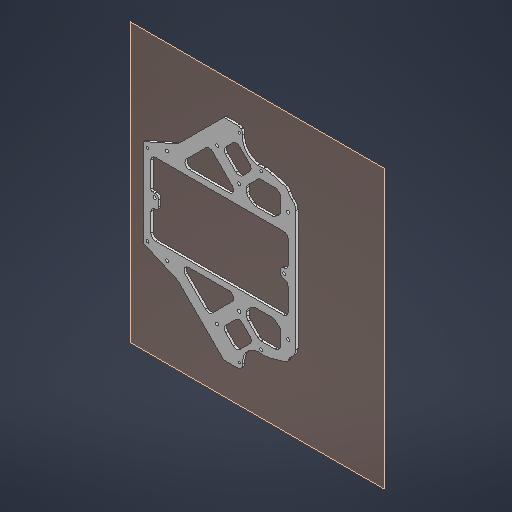
# Autodesk Inventor part: NewBody
Saved by Autodesk Inventor 2026.1 (Build 301233020, 233B)
## iProperties
Created: 2026-01-11
Part Number: NewBody
Material: 一般
Document SubType Name: Modeling
Designer: kamada
Density: 1 g/cm^3
Appearance: 既定
Author: kamada
Autodesk Inventor part; units mm, degrees
(part 1 of 2)
ref_plane "YZ Plane" through (0, 0, 0) normal (1, 0, 0) x (0, 1, 0)
ref_plane "XZ Plane" through (0, 0, 0) normal (0, 1, 0) x (-1, 0, 0)
ref_plane "XY Plane" through (0, 0, 0) normal (0, 0, 1) x (1, 0, 0)
ref_plane "作業平面1" through (0, 0, 0) normal (0, 0, 1) x (1, 0, 0)
sketch "スケッチ1" plane through (0, 0, 0) normal (0, 0, 1) x (1, 0, 0)
  line L0 (95, 63.3506) -> (95, -15.777) projected
  ellipse E0 centre (89, -15.777) end of major axis (89, -21.777) minor radius 6 (93.618, -19.6078) -> (95, -15.777) ccw projected
  ellipse E1 centre (89, -15.777) end of major axis (83, -15.777) minor radius 6 (92.5, -20.6504) -> (93.618, -19.6078) ccw projected
  ellipse E2 centre (96, -25.5238) end of major axis (90, -25.5238) minor radius 6 (92.5, -20.6504) -> (90, -25.5238) ccw projected
  line L1 (90, -40.6801) -> (90, -25.5238) projected
  line L2 (71.7064, -58.9737) -> (90, -40.6801) projected
  line L3 (61.6653, -58.9737) -> (71.7064, -58.9737) projected
  line L4 (7.6928, -5.0012) -> (61.6653, -58.9737) projected
  circle A0 centre (43.3868, -26.8548) radius 1.05 projected
  circle A1 centre (57.8825, -12.3591) radius 1.05 projected
  circle A2 centre (72.5196, -26.9962) radius 1.05 projected
  circle A3 centre (57.8825, 59.9352) radius 1.05 projected
  circle A4 centre (43.3868, 74.4309) radius 1.05 projected
  circle A5 centre (72.5196, 74.5724) radius 1.05 projected
  ellipse E3 centre (89, 63.3506) end of major axis (89, 69.3506) minor radius 6 (95, 63.3506) -> (92.5, 68.224) ccw projected
  ellipse E4 centre (96, 73.0974) end of major axis (96, 79.0974) minor radius 6 (90, 73.0974) -> (92.5, 68.224) ccw projected
  line L5 (90, 88.2549) -> (90, 73.0974) projected
  line L6 (71.7064, 106.5485) -> (90, 88.2549) projected
  line L7 (61.6653, 106.5485) -> (71.7064, 106.5485) projected
  line L8 (7.6928, 52.576) -> (61.6653, 106.5485) projected
  line L9 (90, 52.5748) -> (-5, 52.5748) projected
  line L10 (-5, 36.1871) -> (-5, 52.5748) projected
  line L11 (-5, 32.971) -> (-5, 36.1873) projected
  line L12 (-5, 30.2874) -> (-5, 32.971) projected
  line L13 (-5, 17.2874) -> (-5, 30.2874) projected
  line L14 (-5, 14.6035) -> (-5, 17.2874) projected
  line L15 (-5, 11.3873) -> (-5, 14.6035) projected
  line L16 (-5, 11.3871) -> (-5, -5.0012) projected
  line L17 (0, -5) -> (90, -5) projected
  line L18 (7.6928, -5.0012) -> (-5, -5.0012) projected
  line L19 (53.5082, 23.0012) -> (5, 23.0012) projected
  line L20 (53.5082, 24.5012) -> (53.5082, 23.0012) projected
  ellipse E5 centre (57.0082, 24.5012) end of major axis (53.5082, 24.5012) minor radius 3.5 (60.5082, 24.5012) -> (53.5082, 24.5012) ccw projected
  line L21 (60.5082, 18.2012) -> (60.5082, 24.5012) projected
  line L22 (0, 18.2012) -> (60.5082, 18.2012) projected
  line L23 (0, 18.2012) -> (0, 0) projected
  line L24 (90, 0) -> (0, 0) projected
  line L25 (90, 0) -> (90, 47.576) projected
  line L26 (0, 47.576) -> (90, 47.576) projected
  line L27 (0, 47.576) -> (0, 28.0012) projected
  arc A6 (0, 28.0012) -> (1, 27.0012) centre (1, 28.0012) ccw projected
  line L28 (1, 27.0012) -> (2.5, 27.0012) projected
  ellipse E6 centre (2.5, 24.5012) end of major axis (5, 24.5012) minor radius 2.5 (5, 24.5012) -> (2.5, 27.0012) ccw projected
  line L29 (5, 24.5012) -> (5, 23.0012) projected
  line L30 (87, 20.7876) -> (87, 22.9055) projected
  circle A7 centre (87.471, 23.7874) radius 1 projected
  ellipse E7 centre (87.471, 23.7874) end of major axis (84.4343, 23.7874) minor radius 3.0367 (85, 22.0222) -> (87, 20.7874) ccw projected
  arc A8 (90, 17.7874) -> (87, 20.7874) centre (87, 17.7874) ccw projected
  line L31 (90, 26.7874) -> (90, 17.7874) projected
  line L32 (90, 26.7874) -> (87, 26.7874) projected
  ellipse E8 centre (87.471, 23.7874) end of major axis (84.4343, 23.7874) minor radius 3.0367 (87, 26.7874) -> (85, 25.5526) ccw projected
  line L33 (85, 22.0222) -> (85, 25.5526) projected
  ellipse E9 centre (87, 29.7874) end of major axis (87, 32.7874) minor radius 3 (87, 26.7874) -> (90, 29.7874) ccw projected
  line L34 (90, 47.5748) -> (90, 52.5748) projected
  line L35 (90, -20.2311) -> (90, 0) projected
  circle A9 centre (72.5196, 74.5724) radius 1.05 projected
  circle A10 centre (43.3868, 74.4309) radius 1.05 projected
  circle A11 centre (57.8825, 59.9352) radius 1.05 projected
  line L36 (74.0275, 76.9631) -> (69.9975, 76.6465) projected
  line L37 (69.9975, 76.6465) -> (64.2656, 70.9146) projected
  line L38 (64.2656, 70.9146) -> (47.9538, 82.5385) projected
  line L39 (47.9538, 82.5385) -> (37.0141, 71.5988) projected
  line L40 (37.0141, 71.5988) -> (55.3316, 53.2813) projected
  line L41 (55.3316, 53.2813) -> (78.0106, 76.3832) projected
  line L42 (78.0106, 76.3832) -> (74.0275, 76.9631) projected
  circle A12 centre (72.5196, -26.9962) radius 1.05 projected
  circle A13 centre (43.3868, -26.8548) radius 1.05 projected
  circle A14 centre (57.8825, -12.3591) radius 1.05 projected
  line L43 (64.2656, -23.3385) -> (47.9538, -34.9624) projected
  line L44 (70.0856, -29.1585) -> (64.2656, -23.3385) projected
  ellipse E10 centre (71.1407, -40.1131) end of major axis (82.146, -40.1131) minor radius 11.0053 (73.7648, -29.4252) -> (70.0856, -29.1585) ccw projected
  line L45 (78.0106, -28.8071) -> (73.7648, -29.4252) projected
  line L46 (55.3316, 53.2813) -> (85.5, 84.0122) projected
  line L47 (85.5, 84.0122) -> (85.5, 88.2549) projected
  line L48 (85.5, 88.2549) -> (71.7064, 102.0485) projected
  line L49 (71.7064, 102.0485) -> (67.4638, 102.0485) projected
  line L50 (67.4638, 102.0485) -> (37.0141, 71.5988) projected
  arc A15 (90, -13.4106) -> (90, -11.3106) centre (89.9988, -12.3606) ccw projected
  line L51 (90, -19.6078) -> (90, -13.4106) projected
  line L52 (93.618, -19.6078) -> (90, -19.6078) projected
  ellipse E11 centre (89, -15.777) end of major axis (89, -21.777) minor radius 6 (93.618, -19.6078) -> (95, -15.777) ccw projected
  line L53 (95, 63.3506) -> (95, -15.777) projected
  ellipse E12 centre (89, 63.3506) end of major axis (89, 69.3506) minor radius 6 (95, 63.3506) -> (92.5, 68.224) ccw projected
  ellipse E13 centre (96, 73.0974) end of major axis (96, 79.0974) minor radius 6 (90, 73.0974) -> (92.5, 68.224) ccw projected
  line L54 (90, 88.2549) -> (90, 73.0974) projected
  line L55 (71.7064, 106.5485) -> (90, 88.2549) projected
  line L56 (61.6653, 106.5485) -> (71.7064, 106.5485) projected
  line L57 (7.6928, 52.576) -> (61.6653, 106.5485) projected
  line L58 (7.6928, 52.576) -> (0, 52.576) projected
  line L59 (0, 52.576) -> (0, 52.5748) projected
  line L60 (90, 52.5748) -> (0, 52.5748) projected
  line L61 (90, 47.5748) -> (90, 52.5748) projected
  line L62 (90, 29.7874) -> (90, 47.5748) projected
  ellipse E14 centre (87, 29.7874) end of major axis (87, 32.7874) minor radius 3 (87, 26.7874) -> (90, 29.7874) ccw projected
  line L63 (90, 26.7874) -> (87, 26.7874) projected
  line L64 (90, 0) -> (90, 26.7874) projected
  line L65 (0, 0) -> (90, 0) projected
  line L66 (0, 0) -> (0, -5) projected
  line L67 (0, -5) -> (90, -5) projected
  line L68 (90, -11.3106) -> (90, -5) projected
  circle A16 centre (89.9993, 59.9351) radius 1.05 projected
  line L69 (67.4638, 102.0485) -> (37.0141, 71.5988) projected
  line L70 (71.7064, 102.0485) -> (67.4638, 102.0485) projected
  line L71 (85.5, 88.2549) -> (71.7064, 102.0485) projected
  line L72 (85.5, 84.0122) -> (85.5, 88.2549) projected
  line L73 (55.3316, 53.2813) -> (85.5, 84.0122) projected
  line L74 (37.0141, 71.5988) -> (55.3316, 53.2813) projected
  line L75 (85.5, -36.4374) -> (85.5, -40.6801) projected
  line L76 (71.7064, -54.4737) -> (67.4638, -54.4737) projected
  arc A17 (90, -11.3106) -> (90, -13.4106) centre (89.9988, -12.3606) ccw projected
  line L77 (90, -11.3106) -> (90, -5) projected
  line L78 (90, -5) -> (0, -5) projected
  line L79 (0, 0) -> (0, -5) projected
  line L80 (0, 11.3871) -> (0, 0) projected
  line L81 (0, 11.3871) -> (-5, 11.3871) projected
  line L82 (-5, 11.3871) -> (-5, -5.0012) projected
  line L83 (7.6928, -5.0012) -> (-5, -5.0012) projected
  line L84 (7.6928, -5.0012) -> (61.6653, -58.9737) projected
  line L85 (61.6653, -58.9737) -> (71.7064, -58.9737) projected
  line L86 (71.7064, -58.9737) -> (90, -40.6801) projected
  line L87 (90, -40.6801) -> (90, -25.5238) projected
  ellipse E15 centre (96, -25.5238) end of major axis (90, -25.5238) minor radius 6 (92.5, -20.6504) -> (90, -25.5238) ccw projected
  ellipse E16 centre (89, -15.777) end of major axis (83, -15.777) minor radius 6 (92.5, -20.6504) -> (93.618, -19.6078) ccw projected
  line L88 (90, -19.6078) -> (93.618, -19.6078) projected
  line L89 (90, -19.6078) -> (90, -13.4106) projected
  line L90 (-5, 36.1871) -> (0, 36.1871) projected
  line L91 (0, 36.1871) -> (0, 47.5748) projected
  line L92 (0, 47.5748) -> (90, 47.5748) projected
  line L93 (90, 47.5748) -> (90, 52.5748) projected
  line L94 (90, 52.5748) -> (-5, 52.5748) projected
  line L95 (-5, 36.1871) -> (-5, 52.5748) projected
  line L96 (53.5082, 23.0012) -> (5, 23.0012) projected
  line L97 (53.5082, 24.5012) -> (53.5082, 23.0012) projected
  ellipse E17 centre (57.0082, 24.5012) end of major axis (53.5082, 24.5012) minor radius 3.5 (60.5082, 24.5012) -> (53.5082, 24.5012) ccw projected
  line L98 (60.5082, 18.2012) -> (60.5082, 24.5012) projected
  line L99 (0, 18.2012) -> (60.5082, 18.2012) projected
  line L100 (0, 18.2012) -> (0, 0) projected
  line L101 (90, 0) -> (0, 0) projected
  line L102 (90, 0) -> (90, 47.576) projected
  line L103 (0, 47.576) -> (90, 47.576) projected
  line L104 (0, 47.576) -> (0, 28.0012) projected
  arc A18 (0, 28.0012) -> (1, 27.0012) centre (1, 28.0012) ccw projected
  line L105 (1, 27.0012) -> (2.5, 27.0012) projected
  ellipse E18 centre (2.5, 24.5012) end of major axis (5, 24.5012) minor radius 2.5 (5, 24.5012) -> (2.5, 27.0012) ccw projected
  line L106 (5, 24.5012) -> (5, 23.0012) projected
  line L107 (-5, 36.1871) -> (0, 36.1871) projected
  line L108 (0, 36.1871) -> (0, 47.5748) projected
  line L109 (0, 47.5748) -> (90, 47.5748) projected
  line L110 (90, 47.5748) -> (90, 52.5748) projected
  line L111 (90, 52.5748) -> (-5, 52.5748) projected
  line L112 (-5, 36.1871) -> (-5, 52.5748) projected
  line L113 (7.6935, 52.5766) -> (7.6916, 52.5748)
  line L114 (-5, 11.3873) -> (-5, 11.3871)
  line L115 (7.6931, -5.0015) -> (7.6916, -5)
  line L116 (67.4638, -54.4724) -> (47.9538, -34.9624) projected
  line L117 (47.9538, -34.9624) -> (37.0141, -24.0227) projected
  line L118 (37.0141, -24.024) -> (55.3316, -5.7065) projected
  line L119 (55.3316, -5.7065) -> (85.5, -36.4374) projected
  line L120 (85.5, -40.6788) -> (71.7064, -54.4724) projected
  line L121 (71.7064, -54.4724) -> (67.4638, -54.4724) projected
  point P0 (93.618, -19.6078)
  point P1 (78.0095, -28.8072)
  constraints: 6 end point, 6 point on line, 1 vertical, 20 other
extrude "押し出し1" add sketch "スケッチ1" along normal blind 1.5 contours L0 E0 L52 L35 A15 L25 L34 L9 L8 L7 L6 L5 E4 E3 | E1 E2 L1 L2 L3 L4 L17 L35 A17 L52 | L17 L66 L24 L35 | L9 L34 L26 L27 L90 L10 | L18 L16 L81 L23 L66 | A8 E7 L33 E8 L32 L25 | L81 L15 L14 L13 L12 L11 L90 L27 A6 L28 E6 L29 L19 L20 E5 L21 L22 L23 | L32 E9 L25 | L42 L41 L40 L39 L38 L37 L36 | L43 L117 L118 L119 L45 E10 L44
sketch "スケッチ2" plane through (0, 0, 1.5) normal (0, 0, 1) x (1, 0, 0)
  circle A0 centre (57.0082, 24.5003) radius 1 projected
  circle A1 centre (2.5, 24.5003) radius 1 projected
  point P0 (0, 0)
extrude "押し出し2" cut sketch "スケッチ2" against normal blind 1.5
sketch "スケッチ3" plane through (0, 0, 0) normal (0, 0, -1) x (-1, 0, 0)
  arc A0 (-57.6107, -43.5509) -> (-55.9649, -41.9051) centre (-58.0239, -41.4919) ccw projected
  line L0 (-42.9736, -28.9138) -> (-55.9649, -41.9051) projected
  arc A1 (-42.9736, -28.9138) -> (-41.3278, -27.268) centre (-43.3868, -26.8548) ccw projected
  line L1 (-40.5951, -26.5353) -> (-41.3278, -27.268) projected
  line L2 (-41.7251, -25.4053) -> (-40.5951, -26.5353) projected
  arc A2 (-41.7251, -22.5768) -> (-41.7251, -25.4053) centre (-40.3109, -23.991) ccw projected
  line L3 (-40.5951, -21.4468) -> (-41.7251, -22.5768) projected
  line L4 (-41.585, -20.4569) -> (-40.5951, -21.4468) projected
  line L5 (-60.1861, -39.058) -> (-41.585, -20.4569) projected
  arc A3 (-60.4529, -42.7372) -> (-60.1861, -39.058) centre (-71.1407, -40.1131) ccw projected
  line L6 (-58.6249, -44.5651) -> (-60.4529, -42.7372) projected
  line L7 (-57.6107, -43.5509) -> (-58.6249, -44.5651) projected
  circle A4 centre (-43.3868, -26.8548) radius 0.75 projected
  circle A5 centre (-58.0239, -41.4919) radius 0.75 projected
  line L8 (-41.585, 68.033) -> (-60.1861, 86.6341) projected
  line L9 (-40.5951, 69.0229) -> (-41.585, 68.033) projected
  line L10 (-41.7251, 70.1529) -> (-40.5951, 69.0229) projected
  arc A6 (-41.7251, 72.9814) -> (-41.7251, 70.1529) centre (-40.3109, 71.5672) ccw projected
  line L11 (-40.5951, 74.1114) -> (-41.7251, 72.9814) projected
  line L12 (-41.3278, 74.8441) -> (-40.5951, 74.1114) projected
  arc A7 (-41.3278, 74.8441) -> (-42.9736, 76.4899) centre (-43.3868, 74.4309) ccw projected
  line L13 (-55.9649, 89.4813) -> (-42.9736, 76.4899) projected
  arc A8 (-55.9649, 89.4813) -> (-57.6107, 91.127) centre (-58.0239, 89.068) ccw projected
  line L14 (-58.6249, 92.1412) -> (-57.6107, 91.127) projected
  line L15 (-60.4529, 90.3133) -> (-58.6249, 92.1412) projected
  arc A9 (-60.1861, 86.6341) -> (-60.4529, 90.3133) centre (-71.1407, 87.6892) ccw projected
  circle A10 centre (-58.0239, 89.068) radius 0.75 projected
  circle A11 centre (-43.3868, 74.4309) radius 0.75 projected
  line L16 (-86.7048, 88.7216) -> (-68.878, 106.5485) projected
  line L17 (-86.7048, 77.1384) -> (-86.7048, 88.7216) projected
  line L18 (-79.7466, 78.1515) -> (-86.7048, 77.1384) projected
  line L19 (-79.7466, 78.1515) -> (-85.5, 84.0122) projected
  line L20 (-85.5, 84.0122) -> (-85.5, 88.2549) projected
  line L21 (-85.5, 88.2549) -> (-71.7064, 102.0485) projected
  line L22 (-71.7064, 102.0485) -> (-67.4638, 102.0485) projected
  line L23 (-67.4638, 102.0485) -> (-47.9538, 82.5385) projected
  line L24 (-47.9538, 82.5385) -> (-41.9405, 86.8236) projected
  line L25 (-41.9405, 86.8236) -> (-61.6653, 106.5485) projected
  line L26 (-61.6653, 106.5485) -> (-68.878, 106.5485) projected
  line L27 (-64.2656, 70.9146) -> (-41.9405, 86.8236) projected
  line L28 (-69.9975, 76.6465) -> (-64.636, 71.2849) projected
  line L29 (-64.2656, -23.3378) -> (-41.9405, -39.2473) projected
  line L30 (-68.878, -58.9724) -> (-86.7056, -41.1448) projected
  line L31 (-61.6653, -58.9724) -> (-68.878, -58.9724) projected
  line L32 (-41.9405, -39.2475) -> (-61.6653, -58.9724) projected
  line L33 (-41.9405, -39.2475) -> (-47.9538, -34.9624) projected
  line L34 (-67.4638, -54.4724) -> (-47.9538, -34.9624) projected
  line L35 (-71.7064, -54.4724) -> (-67.4638, -54.4724) projected
  line L36 (-85.5, -40.6788) -> (-71.7064, -54.4724) projected
  line L37 (-85.5, -36.4361) -> (-85.5, -40.6788) projected
  line L38 (-79.7466, -30.5754) -> (-85.5, -36.4361) projected
  line L39 (-86.7056, -29.5622) -> (-79.7466, -30.5754) projected
  line L40 (-86.7056, -41.1448) -> (-86.7056, -29.5622) projected
  line L41 (-60.4529, -42.7372) -> (-58.0907, -45.0993)
  line L42 (-64.636, -23.7082) -> (-64.2656, -23.3378)
  line L43 (-60.4529, 90.3133) -> (-58.0907, 92.6754)
  line L44 (-64.636, 71.2849) -> (-64.2656, 70.9146)
  line L45 (-64.636, 71.2849) -> (-54.3661, 80.8141)
  line L46 (-64.636, -23.7082) -> (-54.7361, -33.608)
  line L47 (-60.3757, -39.2475) -> (-54.7361, -33.608)
  line L48 (-54.7361, -33.608) -> (-64.636, -23.7082)
  line L49 (-70.2755, -29.3477) -> (-60.3757, -39.2475)
  line L50 (-67.4638, -54.4724) -> (-47.9538, -34.9624) projected
  line L51 (-47.9538, -34.9624) -> (-64.2656, -23.3385) projected
  line L52 (-60.1861, -39.058) -> (-52.7049, -31.5767)
  line L53 (-52.7049, -31.5767) -> (-62.6047, -21.6769)
  line L54 (-70.086, -29.1582) -> (-60.1861, -39.058)
  line L55 (-70.0856, -29.1585) -> (-64.2656, -23.3385) projected
  line L56 (-69.9975, 76.6465) -> (-60.1861, 86.6341)
  point P0 (0, 0)
  constraints: 26 end point, 9 point on line, 4 perpendicular, 3 parallel, 1 collinear, 1 point on circle
extrude "押し出し3" add sketch "スケッチ3" against normal up to surface (1.5 mm away) contours L7 L6 A3 L5 L29 L0 A0 | A0 L0 L29 L34 L41 L7 | L5 L46 L42 L29 | L54 L55 L46 L5 | L45 L28 L56 L8 | L8 A9 L15 L14 A8 L13 L27 | L8 L27 L44 L45 | L13 A8 L14 L43 L23 L27
sketch "スケッチ4" plane through (0, 0, 0) normal (0, 0, -1) x (-1, 0, 0)
  circle A0 centre (-71.1407, -40.1131) radius 10 projected
  circle A1 centre (-71.1407, 87.6892) radius 10 projected
  ellipse E0 centre (-71.1407, -40.1131) end of major axis (-60.1355, -40.1131) minor radius 11.0053 (-70.0856, -29.1585) -> (-73.7648, -29.4252) ccw projected
  circle A2 centre (-71.1407, -40.1131) radius 11.0053
  line L0 (-70.0856, -29.1585) -> (-60.1861, -39.058) projected
  line L1 (-60.1861, 86.6341) -> (-69.9975, 76.6465) projected
  circle A3 centre (-71.1407, -40.1131) radius 11.0053
  circle A4 centre (-71.1407, 87.6892) radius 11.1017
  line L2 (-60.1861, 86.6341) -> (-60.0794, 86.7428)
  arc A5 (-60.1861, 86.6341) -> (-60.4529, 90.3133) centre (-71.1407, 87.6892) ccw projected
  line L3 (-58.0907, 92.6754) -> (-60.4529, 90.3133) projected
  point P0 (0, 0)
  point P1 (-68.6682, 77.9997)
  point P2 (-61.4087, 85.3896)
  point P3 (-60.3732, 90.3929)
  constraints: 3 coincident, 3 point on circle, 2 centre point, 2 end point, 4 other
extrude "押し出し4" cut sketch "スケッチ4" against normal up to surface (1.5 mm away) contours L0 A0 | A0 L0 A2 | L1 A1 | A1 L1 L2 A4 | A5 L3 A4 L2 picked at (-64.1383, -34.6551) picked at (-65.57, 80.7173)
fillet "フィレット1" radius 3 4 edges at (0, 47.576, 0.75) (0, 0, 0.75) (90, 47.576, 0.75) (90, 0, 0.75)
sketch "スケッチ5" plane through (0, 0, 0) normal (0, 0, -1) x (-1, 0, 0)
  circle A0 centre (-72.5196, -26.9962) radius 1.05 projected
  circle A1 centre (-58.0239, -41.4919) radius 0.75 projected
  circle A2 centre (-43.3868, -26.8548) radius 1.05 projected
  circle A3 centre (-57.8825, -12.3591) radius 1.05 projected
  circle A4 centre (-72.5196, 74.5724) radius 1.05 projected
  circle A5 centre (-57.8825, 59.9352) radius 1.05 projected
  circle A6 centre (-43.3868, 74.4309) radius 1.05 projected
  circle A7 centre (-58.0239, 89.068) radius 0.75 projected
  line L0 (-72.5196, -26.9962) -> (-58.0239, -41.4919)
  line L1 (-58.0239, -41.4919) -> (-43.3868, -26.8548)
  line L2 (-43.3868, -26.8548) -> (-57.8825, -12.3591)
  line L3 (-57.8825, -12.3591) -> (-72.5196, -26.9962)
  line L4 (-72.5196, 74.5724) -> (-58.0239, 89.068)
  line L5 (-58.0239, 89.068) -> (-43.3868, 74.4309)
  line L6 (-43.3868, 74.4309) -> (-57.8825, 59.9352)
  line L7 (-57.8825, 59.9352) -> (-72.5196, 74.5724)
  line L8 (-67.0029, 72.5912) -> (-57.8825, 63.4708)
  line L9 (-57.8825, 63.4708) -> (-46.9223, 74.4309)
  line L10 (-46.9223, 74.4309) -> (-56.0428, 83.5514)
  line L11 (-56.0428, 83.5514) -> (-67.0029, 72.5912)
  arc A8 (-69.9975, 76.6465) -> (-60.3732, 90.3929) centre (-71.1407, 87.6892) ccw projected
  line L12 (-65.2717, -34.2441) -> (-50.6346, -19.607)
  line L13 (-56.111, -36.0435) -> (-67.0711, -25.0833)
  line L14 (-67.0711, -25.0833) -> (-57.8825, -15.8947)
  line L15 (-57.8825, -15.8947) -> (-46.9223, -26.8548)
  line L16 (-46.9223, -26.8548) -> (-56.111, -36.0435)
  arc A9 (-60.4529, -42.7372) -> (-70.0856, -29.1585) centre (-71.1407, -40.1131) ccw projected
  circle A10 centre (-63.2906, 79.8391) radius 2.5
  point P0 (0, 0)
  point P1 (-63.3588, -32.3312)
  point P2 (-61.5228, 78.0713)
  dimension "d17" = 5
  dimension "d10" = 2.5
  dimension "d12" = 2.5
  dimension "d13" = 2.5
  dimension "d14" = 2.5
  dimension "d15" = 2.5
  dimension "d16" = 2.5
  constraints: 34 end point, 11 parallel, 4 perpendicular, 3 midpoint, 2 point on circle, 2 point on line, 1 coincident, 3 other
  measures "d10" distance between parallel lines of L7 L8
  measures "d12" distance between parallel lines of L9 L6
  measures "d13" distance from line of L13 point (-63.359, -32.331)
  measures "d14" distance between parallel lines of L2 L15
  measures "d15" distance between parallel lines of L3 L14
  measures "d16" distance between parallel lines of L1 L16
extrude "押し出し5" cut sketch "スケッチ5" against normal up to surface (1.5 mm away) contours L13 L14 L15 L12 | L12 L15 L16 L13 | L11 L10 L9 L8
sketch "スケッチ6" plane through (0, 0, 0) normal (0, 0, -1) x (-1, 0, 0)
  line L0 (-7.6928, 52.576) -> (-18.3183, 52.576) projected
  line L1 (-18.3183, -14.9995) -> (-18.3183, 52.576) projected
  line L2 (-18.3183, -14.9995) -> (-17.6928, -14.9995) projected
  line L3 (-7.6928, -4.9997) -> (-17.6928, -14.9995) projected
  line L4 (5, -5) -> (-7.6928, -4.9997) projected
  line L5 (5, 52.576) -> (5, -5) projected
  line L6 (-7.6931, 52.5763) -> (-7.6928, 52.576) projected
  line L7 (-18.3183, 63.2014) -> (-7.6931, 52.5763) projected
  line L8 (-18.3183, 52.576) -> (-18.3183, 63.2014) projected
  line L9 (-7.6928, 52.576) -> (-18.3183, 52.576) projected
  line L10 (-7.6931, 52.5763) -> (-7.6928, 52.576) projected
  line L11 (-17.6928, -14.9995) -> (-17.6928, 62.576)
  line L12 (-7.6916, 52.5748) -> (5, 52.5748) projected
  line L13 (-17.6928, 62.576) -> (5, 52.5748)
  line L14 (-17.6928, -14.9995) -> (5, -5)
  line L15 (-61.6653, 106.5485) -> (-7.6916, 52.5748) projected
  point P0 (0, 0)
  constraints: 6 end point, 1 parallel, 1 point on line
extrude "押し出し6" add sketch "スケッチ6" against normal up to surface (1.5 mm away) contours L7 L13 L12 | L3 L4 L14
sketch "スケッチ7" plane through (0, 0, 0) normal (0, 0, -1) x (-1, 0, 0)
  point P0 (0, 0)
sketch "スケッチ8" plane through (0, 0, 0) normal (0, 0, -1) x (-1, 0, 0)
  line L0 (-67.0711, -25.0833) -> (-57.8825, -15.8947) projected
  line L1 (-57.8825, -15.8947) -> (-46.9223, -26.8548) projected
  line L2 (-46.9223, -26.8548) -> (-56.111, -36.0435) projected
  line L3 (-56.111, -36.0435) -> (-67.0711, -25.0833) projected
  line L4 (-46.9223, 74.4309) -> (-57.8825, 63.4708) projected
  line L5 (-57.8825, 63.4708) -> (-67.0029, 72.5912) projected
  line L6 (-67.0029, 72.5912) -> (-56.0428, 83.5514) projected
  line L7 (-56.0428, 83.5514) -> (-46.9223, 74.4309) projected
  circle A0 centre (-89.9988, -12.3606) radius 1.05 projected
  circle A1 centre (-43.3868, -26.8548) radius 1.05 projected
  circle A2 centre (-57.8825, -12.3591) radius 1.05 projected
  circle A3 centre (-72.5196, -26.9962) radius 1.05 projected
  circle A4 centre (-89.9993, 59.9351) radius 1.05 projected
  arc A5 (-69.9975, 76.6465) -> (-60.3732, 90.3929) centre (-71.1407, 87.6892) ccw projected
  line L8 (-74.0275, 76.9631) -> (-69.9975, 76.6465) projected
  line L9 (-78.0106, 76.3832) -> (-74.0275, 76.9631) projected
  line L10 (-85.5, 84.0122) -> (-78.0106, 76.3832) projected
  line L11 (-85.5, 88.2549) -> (-85.5, 84.0122) projected
  line L12 (-71.7064, 102.0485) -> (-85.5, 88.2549) projected
  line L13 (-67.4638, 102.0485) -> (-71.7064, 102.0485) projected
  line L14 (-58.0907, 92.6754) -> (-67.4638, 102.0485) projected
  line L15 (-58.0907, 92.6754) -> (-60.3732, 90.3929) projected
  circle A6 centre (-87.471, 23.7874) radius 1 projected
  circle A7 centre (-72.5196, 74.5724) radius 1.05 projected
  circle A8 centre (-43.3868, 74.4309) radius 1.05 projected
  circle A9 centre (-57.8825, 59.9352) radius 1.05 projected
  arc A10 (-87, 47.576) -> (-90, 44.576) centre (-87, 44.576) ccw projected
  line L16 (-3, 47.576) -> (-87, 47.576) projected
  arc A11 (0, 44.576) -> (-3, 47.576) centre (-3, 44.576) ccw projected
  line L17 (0, 28.0012) -> (0, 44.576) projected
  arc A12 (-1, 27.0012) -> (0, 28.0012) centre (-1, 28.0012) ccw projected
  line L18 (-2.5, 27.0012) -> (-1, 27.0012) projected
  ellipse E0 centre (-2.5, 24.5012) end of major axis (-5, 24.5012) minor radius 2.5 (-2.5, 27.0012) -> (-5, 24.5012) ccw projected
  line L19 (-5, 23.0012) -> (-5, 24.5012) projected
  line L20 (-53.5082, 23.0012) -> (-5, 23.0012) projected
  line L21 (-53.5082, 24.5012) -> (-53.5082, 23.0012) projected
  ellipse E1 centre (-57.0082, 24.5012) end of major axis (-53.5082, 24.5012) minor radius 3.5 (-53.5082, 24.5012) -> (-60.5082, 24.5012) ccw projected
  line L22 (-60.5082, 18.2012) -> (-60.5082, 24.5012) projected
  line L23 (0, 18.2012) -> (-60.5082, 18.2012) projected
  line L24 (0, 3) -> (0, 18.2012) projected
  arc A13 (-3, 0) -> (0, 3) centre (-3, 3) ccw projected
  line L25 (-87, 0) -> (-3, 0) projected
  arc A14 (-90, 3) -> (-87, 0) centre (-87, 3) ccw projected
  line L26 (-90, 17.7874) -> (-90, 3) projected
  arc A15 (-87, 20.7874) -> (-90, 17.7874) centre (-87, 17.7874) ccw projected
  ellipse E2 centre (-87.471, 23.7874) end of major axis (-84.4343, 23.7874) minor radius 3.0367 (-87, 20.7874) -> (-85, 22.0222) ccw projected
  line L27 (-85, 25.5526) -> (-85, 22.0222) projected
  ellipse E3 centre (-87.471, 23.7874) end of major axis (-84.4343, 23.7874) minor radius 3.0367 (-85, 25.5526) -> (-87, 26.7874) ccw projected
  ellipse E4 centre (-87, 29.7874) end of major axis (-87, 26.7874) minor radius 3 (-90, 29.7874) -> (-87, 26.7874) ccw projected
  line L28 (-90, 44.576) -> (-90, 29.7874) projected
  circle A16 centre (-57.0082, 24.5003) radius 1 projected
  circle A17 centre (-2.5, 24.5003) radius 1 projected
  circle A18 centre (-58.0239, 89.068) radius 0.75 projected
  circle A19 centre (-58.0239, -41.4919) radius 0.75 projected
  arc A20 (-60.4529, -42.7372) -> (-70.0856, -29.1585) centre (-71.1407, -40.1131) ccw projected
  line L29 (-60.4529, -42.7372) -> (-58.0907, -45.0993) projected
  line L30 (-67.4638, -54.4724) -> (-58.0907, -45.0993) projected
  line L31 (-71.7064, -54.4724) -> (-67.4638, -54.4724) projected
  line L32 (-85.5, -40.6788) -> (-71.7064, -54.4724) projected
  line L33 (-85.5, -36.4374) -> (-85.5, -40.6788) projected
  line L34 (-78.0095, -28.8072) -> (-85.5, -36.4374) projected
  line L35 (-73.7648, -29.4252) -> (-78.0095, -28.8072) projected
  ellipse E5 centre (-71.1407, -40.1131) end of major axis (-60.1355, -40.1131) minor radius 11.0053 (-70.0856, -29.1585) -> (-73.7648, -29.4252) ccw projected
  line L36 (5, -5.0012) -> (4.9972, -5.0012) projected
  line L37 (5, 52.5748) -> (5, -5.0012) projected
  line L38 (-61.6653, 106.5485) -> (-17.6928, 62.576) projected
  line L39 (-71.7064, 106.5485) -> (-61.6653, 106.5485) projected
  line L40 (-90, 88.2549) -> (-71.7064, 106.5485) projected
  line L41 (-90, 73.0974) -> (-90, 88.2549) projected
  ellipse E6 centre (-96, 73.0974) end of major axis (-96, 67.0974) minor radius 6 (-92.5, 68.224) -> (-90, 73.0974) ccw projected
  ellipse E7 centre (-89, 63.3506) end of major axis (-89, 69.3506) minor radius 6 (-92.5, 68.224) -> (-95, 63.3506) ccw projected
  line L42 (-95, -15.777) -> (-95, 63.3506) projected
  ellipse E8 centre (-89, -15.777) end of major axis (-83, -15.777) minor radius 6 (-95, -15.777) -> (-92.5, -20.6504) ccw projected
  ellipse E9 centre (-96, -25.5238) end of major axis (-102, -25.5238) minor radius 6 (-90, -25.5238) -> (-92.5, -20.6504) ccw projected
  line L43 (-90, -40.6801) -> (-90, -25.5238) projected
  line L44 (-71.7064, -58.9737) -> (-90, -40.6801) projected
  line L45 (-61.6653, -58.9737) -> (-71.7064, -58.9737) projected
  line L46 (-17.6898, -14.9981) -> (-61.6653, -58.9737) projected
  line L47 (-17.6898, -14.9981) -> (4.9972, -5.0012) projected
  line L48 (-78.0095, -28.8072) -> (-90, -25.5238)
  line L49 (-78.0106, 76.3832) -> (-90, 73.0974)
  line L50 (-58.0907, 92.6754) -> (-47.7923, 92.6754)
  line L51 (-58.0907, -45.0993) -> (-47.791, -45.0993)
  line L52 (5, 52.5748) -> (-17.6928, 62.576) projected
  point P0 (0, 0)
  constraints: 8 end point, 1 horizontal, 1 parallel, 1 point on line, 10 other
extrude "押し出し7" cut sketch "スケッチ8" against normal blind 10 contours L14 L13 L12 L11 L10 L49 L41 L40 L39 L38 L50 | L48 L34 L33 L32 L31 L30 L51 L46 L45 L44 L43
fillet "フィレット2" radius 3 8 edges at (90, -25.5238, 0.75) (90, 73.0974, 0.75) (60.3732, 90.3929, 0.75) (58.0907, 92.6754, 0.75) (47.7923, 92.6754, 0.75) (60.4529, -42.7372, 0.75) (58.0907, -45.0993, 0.75) (47.791, -45.0993, 0.75)
sketch "スケッチ9" plane through (0, 0, 0) normal (0, 0, -1) x (-1, 0, 0)
  line L0 (-41.7934, -20.6653) -> (-51.6929, -10.7658) projected
  line L1 (-51.6929, 58.3419) -> (-41.7934, 68.2414) projected
  line L2 (-58.6249, -45.1335) -> (-40.3109, -26.8195) projected
  line L3 (-55.9649, 89.4813) -> (-42.9736, 76.4899) projected
  line L4 (-58.6249, -45.1335) -> (-13.4914, 0)
  line L5 (-55.9649, 89.4813) -> (-42.9736, 76.4899)
  line L6 (-42.9736, 76.4899) -> (-14.0597, 47.576)
  line L7 (-3, 47.576) -> (-87, 47.576) projected
  line L8 (-13.4914, 0) -> (-14.0597, 47.576)
  line L9 (-54.3418, -8.1169) -> (-37.975, -24.4837)
  line L10 (-37.975, -24.4837) -> (-62.4587, 0)
  line L11 (-38.2592, 71.7756) -> (-62.4588, 47.576)
  line L12 (-62.4587, 0) -> (-62.4588, 47.576)
  line L13 (-87, 0) -> (-3, 0) projected
  line L14 (-62.4587, -4) -> (-13.4914, -4)
  line L15 (-13.4914, -4) -> (-13.4914, 0)
  line L16 (-13.4914, 0) -> (-62.4587, 0)
  line L17 (-62.4587, 0) -> (-62.4587, -4)
  line L18 (-62.4588, 47.576) -> (-14.0597, 47.576)
  line L19 (-14.0597, 47.576) -> (-14.0597, 51.576)
  line L20 (-14.0597, 51.576) -> (-62.4588, 51.576)
  line L21 (-62.4588, 51.576) -> (-62.4588, 47.576)
  point P0 (0, 0)
  point P1 (-45, 0)
  point P2 (-58.4588, 51.576)
  point P3 (-18.0597, 51.576)
  point P4 (-17.4914, -4)
  point P5 (-58.4587, -4)
  dimension "d29" = 4
  dimension "d30" = 4
  constraints: 32 end point, 9 point on line, 4 parallel, 2 horizontal, 2 perpendicular, 1 collinear, 1 midpoint
  measures "d29" distance of L18.end L19.end
  measures "d30" distance of L14.end L4.end
extrude "押し出し8" cut sketch "スケッチ9" against normal blind 10 contours L0 L9 L10 L14 L4 | L20 L11 L1 L6
fillet "フィレット3" radius 3 6 edges at (58.4587, -4, 0.75) (37.975, -24.4837, 0.75) (17.4914, -4, 0.75) (58.4588, 51.576, 0.75) (38.2592, 71.7756, 0.75) (18.0597, 51.576, 0.75)
fillet "フィレット4" radius 3 3 edges at (0, 18.2012, 0.75) (60.5082, 18.2012, 0.75) (53.5082, 23.0012, 0.75)
sketch "スケッチ10" plane through (0, 0, 0) normal (0, 0, -1) x (-1, 0, 0)
  circle A0 centre (-89.9988, -12.3606) radius 1.05 projected
  circle A1 centre (-89.9993, 59.9351) radius 1.05 projected
  circle A2 centre (-57.8825, 59.9352) radius 1.05 projected
  circle A3 centre (-57.8825, -12.3591) radius 1.05 projected
  line L0 (-89.9988, -12.3606) -> (-57.8825, -12.3606)
  line L1 (-57.8825, -12.3606) -> (-57.8825, 59.9352)
  line L2 (-57.8825, 59.9352) -> (-89.9988, 59.9352)
  line L3 (-89.9988, 59.9352) -> (-89.9988, -12.3606)
  line L4 (-87, 0) -> (-3, 0) projected
  line L5 (-89.9988, -12.3606) -> (-57.8825, -12.3606)
  line L6 (-57.8825, -12.3606) -> (-57.8825, 0)
  line L7 (-57.8825, 0) -> (-89.9988, 0)
  line L8 (-89.9988, 0) -> (-89.9988, -12.3606)
  line L9 (-3, 47.576) -> (-87, 47.576) projected
  line L10 (-89.9988, 59.9352) -> (-57.8825, 59.9352)
  line L11 (-57.8825, 59.9352) -> (-57.8825, 47.576)
  line L12 (-57.8825, 47.576) -> (-89.9988, 47.576)
  line L13 (-89.9988, 47.576) -> (-89.9988, 59.9352)
  line L14 (-89.9988, 47.576) -> (-67.0029, 47.576)
  line L15 (-67.0029, 47.576) -> (-67.0029, 72.5912)
  line L16 (-67.0029, 72.5912) -> (-89.9988, 72.5912)
  line L17 (-89.9988, 72.5912) -> (-89.9988, 47.576)
  line L18 (-57.8825, -15.8947) -> (-67.0711, -25.0833) projected
  line L19 (-89.9988, -12.3606) -> (-67.0711, -12.3606)
  line L20 (-67.0711, -12.3606) -> (-67.0711, -25.0833)
  line L21 (-67.0711, -25.0833) -> (-89.9988, -25.0833)
  line L22 (-89.9988, -25.0833) -> (-89.9988, -12.3606)
  line L23 (-89.9988, -25.0833) -> (-67.0711, -25.0833)
  line L24 (-67.0711, -25.0833) -> (-67.0711, -20.0833)
  line L25 (-67.0711, -20.0833) -> (-89.9988, -20.0833)
  line L26 (-89.9988, -20.0833) -> (-89.9988, -25.0833)
  line L27 (-89.9988, 72.5912) -> (-67.0029, 72.5912)
  line L28 (-67.0029, 72.5912) -> (-67.0029, 67.5912)
  line L29 (-67.0029, 67.5912) -> (-89.9988, 67.5912)
  line L30 (-89.9988, 67.5912) -> (-89.9988, 72.5912)
  line L31 (-89.9988, 59.9352) -> (-78.5009, 67.5912)
  line L32 (-78.5009, 67.5912) -> (-57.8825, 59.9352)
  line L33 (-89.9988, -12.3606) -> (-78.535, -20.0833)
  line L34 (-57.8825, -12.3606) -> (-78.535, -20.0833)
  line L35 (-89.9988, -12.3606) -> (-73.9407, 0)
  line L36 (-57.8825, -12.3606) -> (-73.9407, 0)
  line L37 (-89.9988, 47.576) -> (-57.8825, 47.576)
  line L38 (-57.8825, 47.576) -> (-57.8825, 59.9352)
  line L39 (-57.8825, 59.9352) -> (-89.9988, 59.9352)
  line L40 (-89.9988, 59.9352) -> (-89.9988, 47.576)
  line L41 (-89.9988, 59.9352) -> (-73.9407, 47.576)
  line L42 (-57.8825, 59.9352) -> (-73.9407, 47.576)
  line L43 (-89.9988, 47.576) -> (-57.8825, 47.576)
  line L44 (-57.8825, 47.576) -> (-57.8825, 52.576)
  line L45 (-57.8825, 52.576) -> (-89.9988, 52.576)
  line L46 (-89.9988, 52.576) -> (-89.9988, 47.576)
  line L47 (-89.9988, 0) -> (-57.8825, 0)
  line L48 (-57.8825, 0) -> (-57.8825, -5)
  line L49 (-57.8825, -5) -> (-89.9988, -5)
  line L50 (-89.9988, -5) -> (-89.9988, 0)
  line L51 (-57.8825, -15.8947) -> (-62.8825, -15.8947)
  line L52 (-62.8825, -15.8947) -> (-62.8825, 0)
  line L53 (-62.8825, 0) -> (-57.8825, 0)
  line L54 (-57.8825, 0) -> (-57.8825, -15.8947)
  line L55 (-57.8825, 63.4708) -> (-46.9223, 74.4309) projected
  line L56 (-57.8825, 63.4708) -> (-62.8825, 63.4708)
  line L57 (-62.8825, 63.4708) -> (-62.8825, 47.576)
  line L58 (-62.8825, 47.576) -> (-57.8825, 47.576)
  line L59 (-57.8825, 47.576) -> (-57.8825, 63.4708)
  line L60 (-67.0029, 67.5912) -> (-62.8825, 63.4708)
  line L61 (-67.0711, -20.0833) -> (-62.8825, -15.8947)
  line L62 (-89.9988, -25.0833) -> (-84.9988, -25.0833)
  line L63 (-84.9988, -25.0833) -> (-84.9988, 0)
  line L64 (-84.9988, 0) -> (-89.9988, 0)
  line L65 (-89.9988, 0) -> (-89.9988, -25.0833)
  line L66 (-89.9988, 72.5912) -> (-84.9988, 72.5912)
  line L67 (-84.9988, 72.5912) -> (-84.9988, 47.576)
  line L68 (-84.9988, 47.576) -> (-89.9988, 47.576)
  line L69 (-89.9988, 47.576) -> (-89.9988, 72.5912)
  line L70 (-84.9988, 63.2645) -> (-78.535, 72.5912)
  line L71 (-62.8825, 63.4708) -> (-78.535, 72.5912)
  line L72 (-84.9988, -15.7289) -> (-78.535, -25.0833)
  line L73 (-78.535, -25.0833) -> (-62.8825, -15.8947)
  line L74 (-78.535, -25.0833) -> (-84.9988, -20.0833)
  line L75 (-84.9988, 67.5912) -> (-78.535, 72.5912)
  line L76 (-73.9407, 0) -> (-73.9407, -25.0833)
  line L77 (-73.9407, -25.0833) -> (-67.0711, -20.0833)
  line L78 (-73.9407, 47.576) -> (-73.9407, 72.5912)
  line L79 (-73.9407, 72.5912) -> (-67.0029, 67.5912)
  point P0 (0, 0)
  point P1 (-84.9988, 56.087)
  point P2 (-80.4371, 52.576)
  point P3 (-67.4442, 52.576)
  point P4 (-62.8825, 56.087)
  point P5 (-69.954, 67.5912)
  point P6 (-62.8825, -8.5119)
  point P7 (-67.4449, -5)
  point P8 (-80.4364, -5)
  point P9 (-84.9988, -8.5119)
  point P10 (-70.0177, -20.0833)
  dimension "d35" = 5
  dimension "d36" = 5
  dimension "d37" = 5
  dimension "d38" = 5
  dimension "d39" = 5
  dimension "d40" = 5
  dimension "d41" = 5
  dimension "d42" = 5
  constraints: 152 end point, 28 parallel, 25 point on line, 15 perpendicular, 14 horizontal, 5 midpoint
  measures "d35" distance of L24.end L23.end
  measures "d36" distance of L27.end L28.end
  measures "d37" distance of L44.end L43.end
  measures "d38" distance of L47.end L48.end
  measures "d39" distance of L52.end L53.end
  measures "d40" distance of L58.end L57.end
  measures "d41" distance of L64.end L63.end
  measures "d42" distance of L67.end L68.end
extrude "押し出し9" cut sketch "スケッチ10" against normal blind 10 contours L63 L35 L49 L76 L0 | L0 L76 L34 L33 L63 | L72 L25 L63 | L33 L25 L72 | L76 L49 L36 L52 L0 | L0 L20 L34 L76 | L34 L76 L25 | L25 L76 L73 L72 | L25 L72 L74 | L0 L52 L34 L20 | L34 L20 L73 L25 L76 | L25 L73 L76 | L73 L76 L21 | L34 L52 L73 L20 | L73 L20 L25 | L25 L77 L76 L73 | L73 L61 L20 | L41 L67 L2 L78 L45 | L78 L2 L15 L42 L45 | L67 L31 L32 L78 L2 | L70 L29 L31 | L67 L29 L70 | L75 L70 L29 | L78 L32 L15 L2 | L15 L2 L57 L42 | L29 L70 L71 L78 | L29 L78 L32 | L16 L78 L71 | L15 L32 L57 L2 | L78 L29 L71 L15 L32 | L78 L71 L29 | L79 L29 L71 L78 | L15 L71 L57 L32 | L29 L15 L71 | L60 L71 L15
sketch "スケッチ11" plane through (0, 0, 0) normal (0, 0, -1) x (-1, 0, 0)
  line L0 (-67.0711, -25.0833) -> (-57.8825, -15.8947) projected
  line L1 (-67.0711, -20.0833) -> (-73.9407, -25.0833) projected
  line L2 (-73.9407, -25.0833) -> (-60.836, -11.9787)
  line L3 (-62.8825, -15.8947) -> (-67.0711, -20.0833) projected
  line L4 (-62.8825, -8.5119) -> (-62.8825, -15.8947) projected
  line L5 (-73.9407, 72.5912) -> (-67.0029, 67.5912) projected
  line L6 (-73.9407, 72.5912) -> (-59.9752, 58.6258)
  line L7 (-57.8825, 63.4708) -> (-67.0029, 72.5912) projected
  line L8 (-62.8825, 63.4708) -> (-62.8825, 56.087) projected
  line L9 (-67.0029, 67.5912) -> (-62.8825, 63.4708) projected
  point P0 (0, 0)
  point P1 (-62.8825, 61.533)
  point P2 (-62.8825, -14.0251)
  constraints: 4 end point, 2 parallel
extrude "押し出し10" add sketch "スケッチ11" against normal blind 1.5
sketch "スケッチ12" plane through (0, 0, 0) normal (0, 0, -1) x (-1, 0, 0)
  line L0 (-67.4442, 52.576) -> (-80.4371, 52.576) projected
  line L1 (-80.4371, 52.576) -> (-84.9988, 56.087) projected
  line L2 (-84.9988, 56.087) -> (-84.9988, 67.5912) projected
  line L3 (-84.9988, 67.5912) -> (-78.535, 72.5912) projected
  line L4 (-78.535, 72.5912) -> (-73.9407, 72.5912) projected
  line L5 (-73.9407, 72.5912) -> (-62.8825, 61.533) projected
  line L6 (-62.8825, 61.533) -> (-62.8825, 56.087) projected
  line L7 (-62.8825, 56.087) -> (-67.4442, 52.576) projected
  line L8 (-80.4364, -5) -> (-67.4449, -5) projected
  line L9 (-67.4449, -5) -> (-62.8825, -8.5119) projected
  line L10 (-62.8825, -8.5119) -> (-62.8825, -14.0251) projected
  line L11 (-62.8825, -14.0251) -> (-73.9407, -25.0833) projected
  line L12 (-73.9407, -25.0833) -> (-78.535, -25.0833) projected
  line L13 (-78.535, -25.0833) -> (-84.9988, -20.0833) projected
  line L14 (-84.9988, -20.0833) -> (-84.9988, -8.5119) projected
  line L15 (-84.9988, -8.5119) -> (-80.4364, -5) projected
  arc A0 (-49.0336, -45.0993) -> (-46.9123, -44.2207) centre (-49.0336, -42.0993) ccw projected
  line L16 (-17.6898, -14.9981) -> (-46.9123, -44.2207) projected
  line L17 (-17.6898, -14.9981) -> (4.9972, -5.0012) projected
  line L18 (5, -5.0012) -> (4.9972, -5.0012) projected
  line L19 (5, 52.5748) -> (5, -5.0012) projected
  line L20 (5, 52.5748) -> (-17.6928, 62.576) projected
  line L21 (-46.9136, 91.7968) -> (-17.6928, 62.576) projected
  arc A1 (-46.9136, 91.7968) -> (-49.0349, 92.6754) centre (-49.0349, 89.6754) ccw projected
  line L22 (-49.0349, 92.6754) -> (-56.8481, 92.6754) projected
  arc A2 (-56.8481, 92.6754) -> (-58.9694, 91.7968) centre (-56.8481, 89.6754) ccw projected
  line L23 (-58.9694, 91.7968) -> (-59.2623, 91.5038) projected
  arc A3 (-59.2623, 91.5038) -> (-60.1193, 89.0223) centre (-57.141, 89.3825) ccw projected
  arc A4 (-69.9975, 76.6465) -> (-60.1193, 89.0223) centre (-71.1407, 87.6892) ccw projected
  line L24 (-74.0275, 76.9631) -> (-69.9975, 76.6465) projected
  line L25 (-78.0106, 76.3832) -> (-74.0275, 76.9631) projected
  line L26 (-78.0106, 76.3832) -> (-88.1122, 73.6148) projected
  arc A5 (-88.1122, 73.6148) -> (-90.2129, 71.5134) centre (-87.3193, 70.7215) ccw projected
  ellipse E0 centre (-96, 73.0974) end of major axis (-96, 67.0974) minor radius 6 (-92.5, 68.224) -> (-90.2129, 71.5134) ccw projected
  ellipse E1 centre (-89, 63.3506) end of major axis (-89, 69.3506) minor radius 6 (-92.5, 68.224) -> (-95, 63.3506) ccw projected
  line L27 (-95, -15.777) -> (-95, 63.3506) projected
  ellipse E2 centre (-89, -15.777) end of major axis (-83, -15.777) minor radius 6 (-95, -15.777) -> (-92.5, -20.6504) ccw projected
  ellipse E3 centre (-96, -25.5238) end of major axis (-102, -25.5238) minor radius 6 (-90.2129, -23.9396) -> (-92.5, -20.6504) ccw projected
  arc A6 (-90.2129, -23.9396) -> (-88.1117, -26.0409) centre (-87.3194, -23.1474) ccw projected
  line L28 (-88.1117, -26.0409) -> (-78.0095, -28.8072) projected
  line L29 (-73.7648, -29.4252) -> (-78.0095, -28.8072) projected
  ellipse E4 centre (-71.1407, -40.1131) end of major axis (-60.1355, -40.1131) minor radius 11.0053 (-70.0856, -29.1585) -> (-73.7648, -29.4252) ccw projected
  arc A7 (-60.2081, -41.3754) -> (-70.0856, -29.1585) centre (-71.1407, -40.1131) ccw projected
  arc A8 (-60.2081, -41.3754) -> (-59.3492, -43.8408) centre (-57.2279, -41.7195) ccw projected
  line L30 (-59.3492, -43.8408) -> (-58.9694, -44.2207) projected
  arc A9 (-58.9694, -44.2207) -> (-56.8481, -45.0993) centre (-56.8481, -42.0993) ccw projected
  line L31 (-56.8481, -45.0993) -> (-49.0336, -45.0993) projected
  line L32 (-67.0711, -25.0833) -> (-57.8825, -15.8947) projected
  line L33 (-57.8825, -15.8947) -> (-46.9223, -26.8548) projected
  line L34 (-46.9223, -26.8548) -> (-56.111, -36.0435) projected
  line L35 (-56.111, -36.0435) -> (-67.0711, -25.0833) projected
  line L36 (-46.9223, 74.4309) -> (-57.8825, 63.4708) projected
  line L37 (-57.8825, 63.4708) -> (-67.0029, 72.5912) projected
  line L38 (-67.0029, 72.5912) -> (-56.0428, 83.5514) projected
  line L39 (-56.0428, 83.5514) -> (-46.9223, 74.4309) projected
  circle A10 centre (-89.9988, -12.3606) radius 1.05 projected
  circle A11 centre (-43.3868, -26.8548) radius 1.05 projected
  circle A12 centre (-57.8825, -12.3591) radius 1.05 projected
  circle A13 centre (-72.5196, -26.9962) radius 1.05 projected
  circle A14 centre (-89.9993, 59.9351) radius 1.05 projected
  circle A15 centre (-87.471, 23.7874) radius 1 projected
  circle A16 centre (-72.5196, 74.5724) radius 1.05 projected
  circle A17 centre (-43.3868, 74.4309) radius 1.05 projected
  circle A18 centre (-57.8825, 59.9352) radius 1.05 projected
  arc A19 (-60.5082, 21.2012) -> (-57.5082, 18.2012) centre (-57.5082, 21.2012) ccw projected
  line L40 (-3, 18.2012) -> (-57.5082, 18.2012) projected
  arc A20 (0, 15.2012) -> (-3, 18.2012) centre (-3, 15.2012) ccw projected
  line L41 (0, 3) -> (0, 15.2012) projected
  arc A21 (-3, 0) -> (0, 3) centre (-3, 3) ccw projected
  line L42 (-87, 0) -> (-3, 0) projected
  arc A22 (-90, 3) -> (-87, 0) centre (-87, 3) ccw projected
  line L43 (-90, 17.7874) -> (-90, 3) projected
  arc A23 (-87, 20.7874) -> (-90, 17.7874) centre (-87, 17.7874) ccw projected
  ellipse E5 centre (-87.471, 23.7874) end of major axis (-84.4343, 23.7874) minor radius 3.0367 (-87, 20.7874) -> (-85, 22.0222) ccw projected
  line L44 (-85, 25.5526) -> (-85, 22.0222) projected
  ellipse E6 centre (-87.471, 23.7874) end of major axis (-84.4343, 23.7874) minor radius 3.0367 (-85, 25.5526) -> (-87, 26.7874) ccw projected
  ellipse E7 centre (-87, 29.7874) end of major axis (-87, 26.7874) minor radius 3 (-90, 29.7874) -> (-87, 26.7874) ccw projected
  line L45 (-90, 44.576) -> (-90, 29.7874) projected
  arc A24 (-87, 47.576) -> (-90, 44.576) centre (-87, 44.576) ccw projected
  line L46 (-3, 47.576) -> (-87, 47.576) projected
  arc A25 (0, 44.576) -> (-3, 47.576) centre (-3, 44.576) ccw projected
  line L47 (0, 28.0012) -> (0, 44.576) projected
  arc A26 (-1, 27.0012) -> (0, 28.0012) centre (-1, 28.0012) ccw projected
  line L48 (-2.5, 27.0012) -> (-1, 27.0012) projected
  ellipse E8 centre (-2.5, 24.5012) end of major axis (-5, 24.5012) minor radius 2.5 (-2.5, 27.0012) -> (-5, 24.5012) ccw projected
  line L49 (-5, 23.0012) -> (-5, 24.5012) projected
  line L50 (-50.6837, 23.0012) -> (-5, 23.0012) projected
  arc A27 (-53.6027, 25.3089) -> (-50.6837, 23.0012) centre (-50.6837, 26.0012) ccw projected
  ellipse E9 centre (-57.0082, 24.5012) end of major axis (-53.5082, 24.5012) minor radius 3.5 (-53.6027, 25.3089) -> (-60.5082, 24.5012) ccw projected
  line L51 (-60.5082, 21.2012) -> (-60.5082, 24.5012) projected
  circle A28 centre (-57.0082, 24.5003) radius 1 projected
  circle A29 centre (-2.5, 24.5003) radius 1 projected
  circle A30 centre (-58.0239, 89.068) radius 0.75 projected
  circle A31 centre (-58.0239, -41.4919) radius 0.75 projected
  line L52 (-22.6127, -9.1213) -> (-35.8537, -22.3623) projected
  arc A32 (-40.0964, -22.3623) -> (-35.8537, -22.3623) centre (-37.975, -20.241) ccw projected
  line L53 (-40.0964, -22.3623) -> (-53.3374, -9.1213) projected
  arc A33 (-51.2161, -4) -> (-53.3374, -9.1213) centre (-51.2161, -7) ccw projected
  line L54 (-51.2161, -4) -> (-24.734, -4) projected
  arc A34 (-22.6127, -9.1213) -> (-24.734, -4) centre (-24.734, -7) ccw projected
  line L55 (-53.3375, 56.6973) -> (-40.3806, 69.6542) projected
  arc A35 (-36.1379, 69.6542) -> (-40.3806, 69.6542) centre (-38.2592, 67.5329) ccw projected
  line L56 (-36.1379, 69.6542) -> (-23.181, 56.6973) projected
  arc A36 (-25.3023, 51.576) -> (-23.181, 56.6973) centre (-25.3023, 54.576) ccw projected
  line L57 (-25.3023, 51.576) -> (-51.2162, 51.576) projected
  arc A37 (-53.3375, 56.6973) -> (-51.2162, 51.576) centre (-51.2162, 54.576) ccw projected
  line L58 (-78.535, -25.0833) -> (-73.9407, -25.0833)
  line L59 (-73.9407, -25.0833) -> (-73.9407, -22.0833)
  line L60 (-73.9407, -22.0833) -> (-78.535, -22.0833)
  line L61 (-78.535, -22.0833) -> (-78.535, -25.0833)
  line L62 (-82.4133, -22.0833) -> (-70.9407, -22.0833)
  line L63 (-78.535, 72.5912) -> (-73.9407, 72.5912)
  line L64 (-73.9407, 72.5912) -> (-73.9407, 69.5912)
  line L65 (-73.9407, 69.5912) -> (-78.535, 69.5912)
  line L66 (-78.535, 69.5912) -> (-78.535, 72.5912)
  line L67 (-78.535, 69.5912) -> (-82.4133, 69.5912)
  line L68 (-82.4133, 69.5912) -> (-70.6585, 69.5912)
  point P0 (0, 0)
  point P1 (-70.9407, 69.5912)
  dimension "d47" = 3
  dimension "d48" = 3
  constraints: 22 end point, 5 point on line, 4 parallel, 3 horizontal, 2 perpendicular, 1 horizontal alignment, 10 other
  measures "d47" distance of L59.end L58.end
  measures "d48" distance of L63.end L64.end
extrude "押し出し11" add sketch "スケッチ12" against normal blind 1.5 contours L68 L64 L5 | L3 L66 L67 | L64 L65 L66 L4 | L62 L61 L13 | L11 L59 L62 | L61 L60 L59 L12
sketch "スケッチ13" plane through (0, 0, 0) normal (0, 0, -1) x (-1, 0, 0)
  circle A0 centre (-10.5828, -7.3636) radius 1
  circle A1 centre (2.2006, -2.6854) radius 1
  line L0 (-95, -15.777) -> (-95, 63.3506) projected
  line L1 (-95, 23.7868) -> (5, 23.7868)
  line L2 (5, 52.5748) -> (5, -5.0012) projected
  circle A2 centre (-10.5828, 54.9372) radius 1
  circle A3 centre (2.2006, 50.259) radius 1
  point P0 (0, 0)
  dimension "d51" = 2
  dimension "d52" = 2
  constraints: 4 centre point, 2 end point, 2 midpoint, 2 symmetric about line, 2 other
  measures "d51" diameter of A0
  measures "d52" diameter of A1
extrude "押し出し12" cut sketch "スケッチ13" against normal blind 1.5
fillet "フィレット5" radius 3 8 edges at (57.8825, 63.4708, 0.75) (56.0428, 83.5514, 0.75) (46.9223, 74.4309, 0.75) (67.0029, 72.5912, 0.75) (67.0711, -25.0833, 0.75) (57.8825, -15.8947, 0.75) (56.111, -36.0435, 0.75) (46.9223, -26.8548, 0.75)
fillet "フィレット6" radius 3 16 edges at (84.9988, -20.0833, 0.75) (82.4133, -22.0833, 0.75) (84.9988, -8.5119, 0.75) (80.4364, -5, 0.75) (67.4449, -5, 0.75) (62.8825, -8.5119, 0.75) (62.8825, -14.0251, 0.75) (70.9407, -22.0833, 0.75) (67.4442, 52.576, 0.75) (62.8825, 56.087, 0.75) (62.8825, 61.533, 0.75) (70.9407, 69.5912, 0.75) (82.4133, 69.5912, 0.75) (84.9988, 67.5912, 0.75) (84.9988, 56.087, 0.75) (80.4371, 52.576, 0.75)